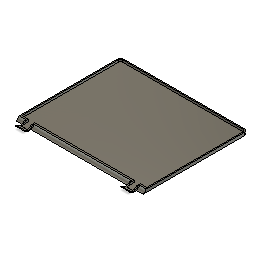
A_case (Autodesk Fusion 360 design; units mm, degrees)
Autodesk Fusion 360 part; units mm, degrees
note: some values were not read from the file. Set by a fixed rule: which sketch regions a step uses.
sketch "Sketch1" plane through (0, 0, 0) normal (0, 1, 0) x (1, 0, 0)
  line L0 (0, 0) -> (230.6, 0)
  line L1 (230.6, 0) -> (230.6, 183)
  line L2 (230.6, 183) -> (0, 183)
  line L3 (0, 183) -> (0, 0)
  dimension "d1" = 230.6
  dimension "d2" = 183
  constraint horizontal L0
  constraint vertical L1
  constraint horizontal L2
  constraint vertical L3
  constraint coincident L0.start L3.end
  measures "d1" distance of L0.start L0.end
  measures "d2" distance of L0.start L2.end
extrude "Extrude1" add sketch "Sketch1" along normal blind 10
sketch "Sketch9" plane through (0, 0, 0) normal (-1, 0, 0) x (0, 0, 1)
  line L0 (-183, 0) -> (0, 0)
  line L1 (0, 0) -> (0, 10)
  line L2 (0, 10) -> (-183, 10)
  line L3 (-183, 10) -> (-183, 0)
  circle A0 centre (11.4881, 10.5) radius 10.5
  line L4 (11.4881, 0) -> (0, 0)
  circle A1 centre (11.4881, 10.5) radius 9
  line L5 (0, 0) -> (1, 0)
  line L6 (1, 0) -> (1, 10)
  line L7 (1, 10) -> (0, 10)
  line L8 (0, 10) -> (0, 0)
  dimension "d69" = 21
  dimension "d70" = 18
  dimension "d94" = 1
  constraint coincident A0 L4.start
  constraint coincident L0.end L1.start
  constraint tangent A0 L4
  constraint parallel L0 L4
  constraint concentric A0 A1
  constraint horizontal L5
  constraint vertical L6
  constraint horizontal L7
  constraint vertical L8
  constraint coincident A0 L6.end
  constraint collinear L2 L7
  measures "d69" diameter of A0
  measures "d70" diameter of A1
  measures "d94" distance of L0.end L5.end
extrude "Extrude8" add sketch "Sketch9" against normal up to surface (230.6 mm away) contours L1 L4 L5 L6 L7 L8 | A0 L4 L6 | A0
sketch "Sketch10" plane through (0, 0, 0) normal (0, -1, 0) x (1, 0, 0)
  line L0 (230.6, -183) -> (230.6, 11.4881)
  line L1 (230.6, 11.4881) -> (0, 11.4881)
  line L2 (0, 11.4881) -> (0, -183)
  line L3 (230.6, 0) -> (218.6, 0)
  line L4 (218.6, 0) -> (218.6, 22)
  line L5 (218.6, 22) -> (230.6, 22)
  line L6 (230.6, 22) -> (230.6, 0)
  line L7 (203.6, 0) -> (27, 0)
  line L8 (27, 0) -> (27, 22)
  line L9 (27, 22) -> (203.6, 22)
  line L10 (203.6, 22) -> (203.6, 0)
  line L11 (0, 0) -> (12, 0)
  line L12 (12, 0) -> (12, 22)
  line L13 (12, 22) -> (0, 22)
  line L14 (0, 22) -> (0, 0)
  line L15 (0, -183) -> (230.6, -183)
  dimension "d73" = 22
  dimension "d74" = 12
  dimension "d75" = 12
  dimension "d76" = 15
  dimension "d77" = 15
  constraint vertical L4
  constraint horizontal L5
  constraint vertical L6
  constraint horizontal L7
  constraint vertical L8
  constraint horizontal L9
  constraint vertical L10
  constraint horizontal L11
  constraint vertical L12
  constraint horizontal L13
  constraint vertical L14
  constraint coincident L11.start L14.end
  constraint collinear L5 L9
  constraint collinear L9 L13
  constraint collinear L0 L6
  constraint parallel L1 L3
  constraint collinear L3 L7
  constraint collinear L7 L11
  measures "d73" distance of L3.start L5.end
  measures "d74" distance of L3.start L3.end
  measures "d75" distance of L12.end L13.end
  measures "d76" distance of L8 L12
  measures "d77" distance of L4 L10
extrude "Extrude9" cut sketch "Sketch10" against normal through all contours L0 L1 L3 L4 L6 | L1 L4 L5 L6 | L1 L2 L11 L12 L14 | L1 L12 L13 L14 | L1 L7 L8 L10 | L1 L8 L9 L10
sketch "Sketch11" plane through (0, 10, 0) normal (0, 1, 0) x (-1, 0, 0)
  line L0 (0, -183) -> (0, 0)
  line L1 (-1.8, -176) -> (-228.8, -176)
  line L2 (-228.8, -176) -> (-228.8, -1)
  line L3 (-228.8, -1) -> (-1.8, -1)
  line L4 (-1.8, -1) -> (-1.8, -176)
  line L5 (-115.3, -122.9084) -> (-115.3, -50) construction
  line L6 (-230.6, 0) -> (-230.6, -183)
  line L7 (-230.6, -183) -> (0, -183)
  line L8 (-12, 0) -> (-12, 1)
  line L9 (-12, 1) -> (-27, 1)
  line L10 (-27, 1) -> (-27, 0)
  line L11 (-27, 0) -> (-203.6, 0)
  line L12 (-203.6, 0) -> (-203.6, 1)
  line L13 (-203.6, 1) -> (-218.6, 1)
  line L14 (-218.6, 1) -> (-218.6, 0)
  line L15 (-218.6, 0) -> (-230.6, 0)
  line L16 (0, 0) -> (-12, 0)
  dimension "d79" = 227
  dimension "d80" = 175
  constraint horizontal L1
  constraint vertical L2
  constraint horizontal L3
  constraint vertical L4
  constraint symmetric L2 L4 L5
  measures "d79" distance of L1.start L1.end
  measures "d80" distance of L1.start L3.end
extrude "Extrude10" cut sketch "Sketch11" against normal blind 2 contours L1 L2 L3 L4
sketch "Sketch12" plane through (0, 8, 0) normal (0, 1, 0) x (-1, 0, 0)
  line L0 (-1.8, -1) -> (-228.8, -1)
  line L1 (-1.8, -176) -> (-1.8, -1)
  line L2 (-6.95, -6.345) -> (-223.65, -6.345)
  line L3 (-223.65, -6.345) -> (-223.65, -181.345)
  line L4 (-223.65, -181.345) -> (-6.95, -181.345)
  line L5 (-6.95, -181.345) -> (-6.95, -6.345)
  line L6 (-10.47, -167.125) -> (-220.13, -167.125)
  line L7 (-220.13, -167.125) -> (-220.13, -9.875)
  line L8 (-220.13, -9.875) -> (-10.47, -9.875)
  line L9 (-10.47, -9.875) -> (-10.47, -167.125)
  line L10 (-85, -88.5) -> (-145, -88.5) construction
  line L11 (-115.3, -115.3819) -> (-115.3, -64.9996) construction
  line L12 (-228.8, -1) -> (-228.8, -176)
  line L13 (-228.8, -176) -> (-1.8, -176)
  dimension "d84" = 175
  dimension "d85" = 216.7
  dimension "d86" = 209.66
  dimension "d87" = 157.25
  dimension "d88" = 3.52
  dimension "d89" = 3.53
  constraint horizontal L2
  constraint vertical L3
  constraint horizontal L4
  constraint vertical L5
  constraint horizontal L6
  constraint vertical L7
  constraint horizontal L8
  constraint vertical L9
  constraint parallel L3 L11
  constraint symmetric L7 L9 L11
  constraint symmetric L6 L8 L10
  measures "d84" distance of L2.start L4.end
  measures "d85" distance of L3.end L4.end
  measures "d86" distance of L6.start L6.end
  measures "d87" distance of L6.start L8.end
  measures "d88" distance of L5 L9
  measures "d89" distance of L2 L8
extrude "Extrude11" cut sketch "Sketch12" against normal blind 1 contours L2 L3 L5 L13 | L3 L4 L5 L13 | L6 L7 L8 L9
fillet "Fillet1" radius 6 2 edges at (0, 5, -183) (230.6, 5, -183)
sketch "Sketch15" plane through (12, 0, 0) normal (-1, 0, 0) x (0, 0, 1)
  line L0 (0, 10) -> (0, 0)
  line L1 (0, 0) -> (11.4881, 0)
  arc A0 (11.4881, 0) -> (1, 10) centre (11.4881, 10.5) ccw
  circle A1 centre (11.4881, 10.5) radius 11.499
  line L2 (0, 0) -> (6.8002, 0)
  line L3 (1, 10) -> (0, 10)
  circle A2 centre (11.4881, 10.5) radius 9
  constraint coincident L0.start A1
  constraint coincident L0.end L1.start
  constraint coincident L1 L2.end
  constraint coincident A1 L2.end
  constraint coincident A0.centre A1.centre
extrude "Extrude14" add sketch "Sketch15" along normal blind 12 and the other way blind 218.6 contours L0 L1 A1 L2
sketch "Sketch13" plane through (0, 0, 0) normal (-1, 0, 0) x (0, 0, 1)
  line L0 (-177, 10) -> (-177, 0)
  line L1 (-177, 0) -> (6.8002, 0)
  line L2 (0, 10) -> (-177, 10)
  line L3 (-183, 5.4) -> (22, 5.4)
  line L4 (22, 5.4) -> (22, 23.4)
  line L5 (22, 23.4) -> (-183, 23.4)
  line L6 (-183, 23.4) -> (-183, 5.4)
  arc A0 (0, 10) -> (6.8002, 0) centre (11.4881, 10.5) ccw
  dimension "d95" = 4.6
  dimension "d96" = 6
  dimension "d97" = 205
  dimension "d98" = 18
  constraint horizontal L3
  constraint vertical L4
  constraint horizontal L5
  constraint vertical L6
  measures "d95" distance of L2 L3
  measures "d96" distance of L0 L6
  measures "d97" distance of L4.end L5.end
  measures "d98" distance of L3.start L5.end
extrude "Extrude12" cut sketch "Sketch13" against normal through all contours L0 L2 L3 A0 | L0 L2 L3 L4 L5 L6 A0
sketch "Sketch14" plane through (0, 5.4, 0) normal (0, 1, 0) x (-1, 0, 0)
  arc A0 (-6, -183) -> (0, -177) centre (-6, -177) ccw
  line L0 (0, -177) -> (0, 1.182)
  line L1 (-12, 1.182) -> (-12, 4.0726)
  line L2 (-12, 4.0726) -> (-27, 4.0726)
  line L3 (-27, 4.0726) -> (-27, 1.182)
  line L4 (-203.6, 1.182) -> (-203.6, 4.0726)
  line L5 (-203.6, 4.0726) -> (-218.6, 4.0726)
  line L6 (-218.6, 4.0726) -> (-218.6, 1.182)
  line L7 (-230.6, 1.182) -> (-230.6, -177)
  arc A1 (-230.6, -177) -> (-224.6, -183) centre (-224.6, -177) ccw
  line L8 (-224.6, -183) -> (-6, -183)
  line L9 (-2, -177) -> (-2, -2)
  line L10 (-2, -2) -> (-14, -2)
  line L11 (-14, -2) -> (-14, 2.0726)
  line L12 (-14, 2.0726) -> (-25, 2.0726)
  line L13 (-25, 2.0726) -> (-25, -2)
  line L14 (-25, -2) -> (-205.6, -2)
  line L15 (-205.6, -2) -> (-205.6, 2.0726)
  line L16 (-205.6, 2.0726) -> (-216.6, 2.0726)
  line L17 (-216.6, 2.0726) -> (-216.6, -2)
  line L18 (-216.6, -2) -> (-228.6, -2)
  line L19 (-228.6, -2) -> (-228.6, -177)
  arc A2 (-228.6, -177) -> (-224.6, -181) centre (-224.6, -177) ccw
  line L20 (-224.6, -181) -> (-6, -181)
  arc A3 (-6, -181) -> (-2, -177) centre (-6, -177) ccw
  line L21 (-14, 2.0726) -> (-25, 2.0726)
  line L22 (-25, 2.0726) -> (-25, 11.5726)
  line L23 (-25, 11.5726) -> (-14, 11.5726)
  line L24 (-14, 11.5726) -> (-14, 2.0726)
  line L25 (-205.6, 2.0726) -> (-216.6, 2.0726)
  line L26 (-216.6, 2.0726) -> (-216.6, 11.5726)
  line L27 (-216.6, 11.5726) -> (-205.6, 11.5726)
  line L28 (-205.6, 11.5726) -> (-205.6, 2.0726)
  line L29 (-27, 1.182) -> (-203.6, 1.182)
  line L30 (-218.6, 1.182) -> (-230.6, 1.182)
  line L31 (0, 1.182) -> (-12, 1.182)
  dimension "d101" = 9.5
  dimension "d102" = 9.5
  constraint horizontal L21
  constraint vertical L22
  constraint horizontal L23
  constraint vertical L24
  constraint collinear L13 L22
  constraint horizontal L25
  constraint vertical L26
  constraint horizontal L27
  constraint vertical L28
  constraint collinear L17 L26
  constraint parallel L0 L9
  constraint parallel L1 L11
  constraint parallel L2 L12
  constraint parallel L3 L13
  constraint parallel L4 L15
  constraint parallel L5 L16
  constraint parallel L6 L17
  constraint parallel L7 L19
  constraint concentric A1 A2
  constraint parallel L8 L20
  constraint concentric A0 A3
  constraint tangent A2 L20
  constraint tangent L19 A2
  constraint tangent L20 A3
  constraint tangent L9 A3
  measures "d101" distance of L11.end L23.end
  measures "d102" distance of L15.end L27.end
extrude "Extrude13" cut sketch "Sketch14" against normal blind 3.9 contours L2 L12 L21 L22 L24 | L2 L22 L23 L24 | L9 L10 L11 L12 L13 L14 L15 L16 L17 L18 L19 A2 L20 A3 L21 L25 | L5 L26 L27 L28 | L5 L16 L25 L26 L28
